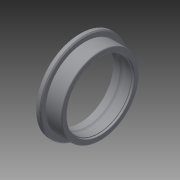
# Autodesk Inventor part: RF-2210X2HH_or
Saved by Autodesk Inventor 2014 SP2 (Build 180246200, 246)
## iProperties
Created: 2019-07-25
Part Number: RF-2210X2HH_or
Material: Generic
Catalog Web Link: www.cadenas.de
Description: Radial Flanged Ball Bearings (RF-Series/LF series) Metric ST or-Radial Flanged Ball Bearings (RF-Series/LF series) Metric Shielded Type
Vendor: NMB
Document SubType Name: Modeling
Designer: psadmin
Manufacturer: NMB
Mass: 0.763578 g
Surface Area: 11.7986 cm^2
Volume: 0.763578 cm^3
Density: 1 g/cm^3
Appearance: PSOLRGB-192-192-192
Category: PARTsolutions
Company: NMB
Title: RF-2210X2HH_or
Author: Cadenas PARTsolutions
Comments: Radial Flanged Ball Bearings (RF-Series/LF series) Metric Shielded Type
PSOL_IDENT_0: {$CADENAS_DATA\23d-libs\nmb\pbbp\radial_flanged_ball_bearings\rfbb_rflfs_m\rflf_shielded_or.prj},227
PSOL_IDENT_1: {VTYP=3D},{NB=RF-2210X2HH_or},{LINA=RF-2210X2HH_or},{NN=Radial Flanged Ball Bearings (RF-Series/LF
PSOL_IDENT_2: series) Metric ST or},{DATE=11.11.2013 05:13:45},{GEOMDATE=24.10.2013 13:34:00},{VERSION=},{LINEID=1
PSOL_IDENT_3: 560},{WBVAR=},{WBNUMERIC=}  {NB=RF-2210X2HH_or},{LINA=RF-2210X2HH_or},{KT=DUMMY},{IDNR=},{PN=RF-2210
PSOL_IDENT_4: X2HH},{SHLD=shielded},{FLANG=flanged},{SD=10.000},{D=22.000},{B=6.000},{SR=0.30},{BCZ=9},{DW=3.1750}
PSOL_IDENT_5: ,{LI=12.40},{LO=19.08},{D1=25.000},{C1=1.50},{D2=0.0},{C2=0.00},{COR=1273},{CR=1065},{PCD=16.000},{U=
PSOL_IDENT_6: 19.175},{W=12.825},{Y=1.588},{Z=1.588},{AA=18.858},{AC=1.20},{AD=0.000},{AF=0.00},{AQ=0.20},{AH=19.2
PSOL_IDENT_7: 8},{AI=12.60},{AJ=0.40}
NN: Radial Flanged Ball Bearings (RF-Series/LF series) Metric ST or
NT: Radial Flanged Ball Bearings (RF-Series/LF series) Metric Shielded Type
NB: RF-2210X2HH_or
NBSYN: $PN._or
LINA: RF-2210X2HH_or
PN: RF-2210X2HH
SHLD: shielded
FLANG: flanged
SD: 10
D: 22
B: 6
SR: 0.3
BCZ: 9
DW: 3.175
LI: 12.4
LO: 19.08
D1: 25
C1: 1.5
D2: 0
C2: 0
COR: 1273
CR: 1065
PCD: 16
U: 19.175
W: 12.825
Y: 1.588
Z: 1.588
AA: 18.858
AC: 1.2
AD: 0
AF: 0
AQ: 0.2
AH: 19.28
AI: 12.6
AJ: 0.4
SUPPLIER: NMB
ARTICLENO: RF-2210X2HH_or
BOMINFO: RF-2210X2HH_or
CREATOR: CADENAS GmbH
Autodesk Inventor part; units mm, degrees
ref_plane "YZ Plane" through (0, 0, 0) normal (1, 0, 0) x (0, 1, 0)
ref_plane "XZ Plane" through (0, 0, 0) normal (0, 1, 0) x (-1, 0, 0)
ref_plane "XY Plane" through (0, 0, 0) normal (0, 0, 1) x (1, 0, 0)
sketch "Sketch_3" plane through (0, 0, 0) normal (0, 0, 1) x (1, 0, 0)
  line L0 (5.7, 0) -> (0, 0)
  line L1 (0, 12.2) -> (0, 9.69)
  arc A0 (0, 9.69) -> (0.15, 9.54) centre (0.15, 9.69) ccw
  line L2 (0.15, 9.54) -> (0.605, 9.54)
  line L3 (0.605, 9.54) -> (0.605, 9.3335)
  line L4 (0.605, 9.3335) -> (2.1386, 9.3335)
  arc A1 (3.8614, 9.3335) -> (2.1386, 9.3335) centre (3, 8) ccw
  line L5 (3.8614, 9.3335) -> (5.4, 9.3335)
  line L6 (5.4, 9.3335) -> (5.4, 9.54)
  line L7 (5.4, 9.54) -> (5.85, 9.54)
  arc A2 (5.85, 9.54) -> (6, 9.69) centre (5.85, 9.69) ccw
  line L8 (6, 9.69) -> (6, 10.7)
  arc A3 (6, 10.7) -> (5.7, 11) centre (5.7, 10.7) ccw
  line L9 (5.7, 11) -> (1.5, 11)
  line L10 (1.5, 11) -> (1.5, 12.2)
  line L11 (1.5, 12.2) -> (1.2, 12.5)
  line L12 (1.2, 12.5) -> (0.3, 12.5)
  line L13 (0.3, 12.5) -> (0, 12.2)
  constraints: 28 end point, 8 point on circle, 4 centre point
revolve "Revolution1" add sketch "Sketch_3" angle 360 about axis through (5.7, 0, 0) along (1, 0, 0)
ref_plane "1_XY" through (3, 0, 0) normal (1, 0, 0) x (0, 0, -1)
ref_plane "1_YZ" through (3, 0, 0) normal (0, 0, -1) x (0, 1, 0)
ref_plane "1_ZX" through (3, 0, 0) normal (0, 1, 0) x (1, 0, 0)
body "Solid1"
